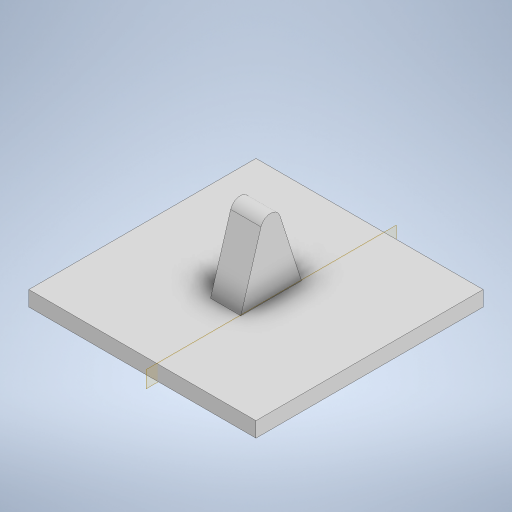
# Autodesk Inventor part: servo-mount
Saved by Autodesk Inventor 2023 (Build 270158000, 158)
## iProperties
Created: 2023-01-30
Part Number: servo-mount
Material: Generic
Document SubType Name: Modeling
Designer: ringl
Density: 1 g/cm^3
Appearance: Default
Author: ringl
Autodesk Inventor part; units mm, degrees
ref_plane "YZ Plane" through (0, 0, 0) normal (1, 0, 0) x (0, 1, 0)
ref_plane "XZ Plane" through (0, 0, 0) normal (0, 1, 0) x (-1, 0, 0)
ref_plane "XY Plane" through (0, 0, 0) normal (0, 0, 1) x (1, 0, 0)
sketch "Sketch1" plane through (0, 0, 0) normal (0, 1, 0) x (-1, 0, 0)
  line L0 (0, 0) -> (30, 0)
  line L1 (30, 0) -> (30, -30)
  line L2 (30, -30) -> (0, -30)
  line L3 (0, -30) -> (0, 0)
  dimension "d0" = 30
  dimension "d1" = 30
  constraints: 8 end point, 2 parallel, 1 horizontal, 1 perpendicular
  measures "d0" distance of L1.end L2.end
  measures "d1" distance of L0.end L1.end
extrude "Extrusion1" add sketch "Sketch1" along normal blind 2
ref_plane "Work Plane1" through (-13, 0, 0) normal (1, 0, 0) x (0, 0, -1)
sketch "Sketch2" plane through (-13, 0, 0) normal (1, 0, 0) x (0, 0, -1)
  line L0 (30, 2) -> (0, 2) projected
  line L1 (19, 2) -> (16.1597, 10.8569)
  line L2 (11, 2) -> (13.6568, 10.8341)
  arc A0 (16.1597, 10.8569) -> (13.6568, 10.8341) centre (14.9118, 10.4567) ccw
  line L3 (0, 0) -> (0, 2) projected
  dimension "d5" = 11
  dimension "d6" = 8
  constraints: 4 end point, 2 point on circle, 2 point on line, 2 tangent, 1 centre point
  measures "d5" distance from line of L3 L2.start
  measures "d6" distance of L2.start L1.start
extrude "Extrusion2" add sketch "Sketch2" against normal blind 4
body "Solid1"
